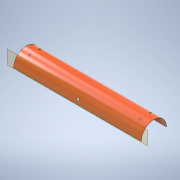
# Autodesk Inventor part: tubo PVC
Saved by Autodesk Inventor 2022 (Build 260153000, 153)
## iProperties
Created: 2022-02-18
Part Number: tubo PVC
Material: Generic
Document SubType Name: Modeling
Designer: Home
Density: 1 g/cm^3
Appearance: Default
Author: Home
Autodesk Inventor part; units mm, degrees
ref_plane "YZ Plane" through (0, 0, 0) normal (1, 0, 0) x (0, 1, 0)
ref_plane "XZ Plane" through (0, 0, 0) normal (0, 1, 0) x (-1, 0, 0)
ref_plane "XY Plane" through (0, 0, 0) normal (0, 0, 1) x (1, 0, 0)
sketch "Sketch1" plane through (0, 0, 0) normal (1, 0, 0) x (0, 1, 0)
  arc A0 (0, -29.8) -> (0, 29.8) centre (0, 0) ccw
  arc A1 (0, -29.48) -> (0, 29.48) centre (0, 0) ccw
  line L0 (0, -29.8) -> (0, -29.48)
  line L1 (0, 29.48) -> (0, 29.8)
  dimension "d0" = 29.8
  dimension "d1" = 59.6
  dimension "d4" = 29.48
  constraints: 4 end point, 4 point on circle, 3 vertical alignment, 2 centre point, 2 coincident, 1 collinear, 1 vertical
  measures "d0" radius of A0
  measures "d1" distance of L1.end L0.start
  measures "d4" radius of A1
extrude "Extrusion1" add sketch "Sketch1" along normal mid plane 300
sketch "Sketch2" plane through (0, 0, 0) normal (0, 0, 1) x (1, 0, 0)
  line L0 (-150, 0) -> (150, 0) projected
  line L1 (-150, 0) -> (150, 0) projected
  line L2 (150, 0) -> (150, 0) projected
  line L3 (150, 0) -> (-150, 0) projected
  line L4 (-150, 0) -> (-150, 0) projected
  point P0 (0, 0)
  point P1 (0, 10)
  point P2 (-134.6305, 7.2182)
  dimension "d7" = 10
  measures "d7" distance from line of L0 point (0, 10)
hole "Hole1" at (0, 10, 0) direction (0, 0, -1) diameter 5.4 end through all both
ref_plane "Work Plane1" through (0, 0, 29.8) normal (0, 0, 1) x (1, 0, 0)
sketch "Sketch3" plane through (0, 0, 29.8) normal (0, 0, 1) x (1, 0, 0)
  line L0 (-150, 29.8) -> (-150, 0) projected
  line L1 (-150, 0) -> (150, 0) projected
  line L2 (150, 0) -> (150, 29.8) projected
  point P0 (0, 0)
  point P1 (-130, 27)
  point P2 (130, 27)
  dimension "d16" = 20
  dimension "d17" = 27
  dimension "d19" = 260
  constraints: 1 horizontal alignment
  measures "d16" distance from line of point (-130, 27) L0
  measures "d17" distance from line of L1 point (-130, 27)
  measures "d19" distance of point (-130, 27) point (130, 27)
hole "Hole2" at (-130, 27, 29.8) at (130, 27, 29.8) direction (0, 0, -1) diameter 2 end through all
body "Solid1"
